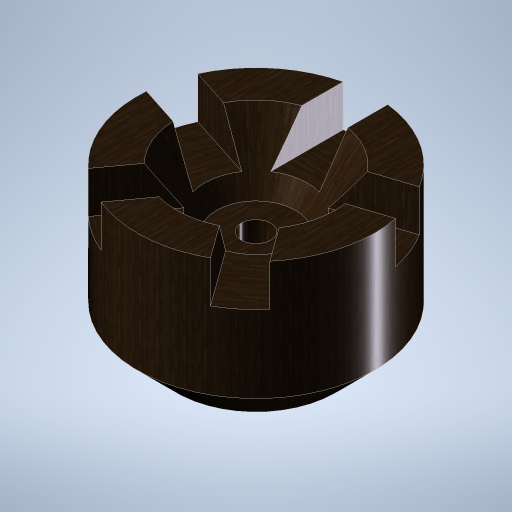
# Autodesk Inventor part: bucket
Saved by Autodesk Inventor 2023 (Build 270158000, 158)
## iProperties
Created: 2023-10-27
Part Number: bucket
Material: Wood (Maple)
Document SubType Name: Modeling
Designer: Admin
Density: 0.67 g/cm^3
Appearance: Natural Maple - Glossy Dark Tint
Author: Admin
Autodesk Inventor part; units mm, degrees
ref_plane "YZ Plane" through (0, 0, 0) normal (1, 0, 0) x (0, 1, 0)
ref_plane "XZ Plane" through (0, 0, 0) normal (0, 1, 0) x (-1, 0, 0)
ref_plane "XY Plane" through (0, 0, 0) normal (0, 0, 1) x (1, 0, 0)
sketch "Sketch1" plane through (0, 0, 0) normal (0, 0, 1) x (1, 0, 0)
  line L0 (-1000, 0) -> (1000, 0)
  line L1 (1000, 0) -> (2000, 1000)
  line L2 (2000, 1000) -> (2000, 4000)
  line L3 (2000, 4000) -> (1000, 4000)
  line L4 (1000, 4000) -> (0, 2500)
  line L5 (0, 2500) -> (-1000, 2500)
  line L6 (-1000, 2500) -> (-1000, 0)
  line L7 (0, 0) -> (1000, 0)
  line L8 (0, 5771.6776) -> (0, -2566.7005)
  dimension "d3" = 3000
  dimension "d4" = 1000
  dimension "d5" = 1000
  dimension "d6" = 1000
  dimension "d7" = 1000
  dimension "d8" = 1000
  dimension "d9" = 1500
  dimension "d19" = 2000
  dimension "d20" = 1000
  constraints: 18 end point, 3 perpendicular, 1 collinear, 1 horizontal, 1 parallel, 1 vertical
  measures "d3" distance of L2.end L1.end
  measures "d4" horizontal distance of L1.end L0.end
  measures "d5" distance of L5.end L4.end
  measures "d6" distance of L2.end L3.end
  measures "d7" horizontal distance of L3.end L4.end
  measures "d8" distance of L7.start L0.end
  measures "d9" vertical distance of L4.end L3.end
  measures "d19" distance from line of L8 L2.end
  measures "d20" distance from line of L8 L0.end
revolve "Revolution1" add sketch "Sketch1" angle 360 mid plane about axis through (-1000, 2500, 0) along (0, -1, 0)
sketch "Sketch2" plane through (-1000, 2500, 0) normal (0, 1, 0) x (1, 0, 0)
  point P0 (1000, 0)
  point P1 (-33.0328, 33.8119)
hole "Hole1" at (-1033.0328, 2500, -33.8119) direction (0, -1, 0) diameter 750 end through all
sketch "Sketch3" plane through (0, 0, 0) normal (1, 0, 0) x (0, 1, 0)
  line L0 (0, -408.8119) -> (2500, -408.8119) projected
  line L1 (1553.7538, -844.1655) -> (1553.7538, 452.6685)
  point P0 (0, 0)
  constraints: 2 end point
sketch "Sketch4" plane through (0, 0, 0) normal (0, 0, 1) x (1, 0, 0)
  line L0 (-1712.8004, 4367.6411) -> (-648.4173, 4367.6411)
  line L1 (-648.4173, 4367.6411) -> (-648.4173, 2948.4636)
  line L2 (-648.4173, 2948.4636) -> (-1712.8004, 2948.4636)
  line L3 (-1712.8004, 2948.4636) -> (-1712.8004, 4367.6411)
  point P0 (0, 0)
  constraints: 8 end point, 2 parallel, 1 horizontal, 1 perpendicular
extrude "Extrusion1" cut sketch "Sketch4" against normal up to next
pattern_circular "Circular Pattern1" count 5 over 360 about axis through (-1000, 3250, 0) along (0, -1, 0) of "Extrusion1"
body "Solid1"
